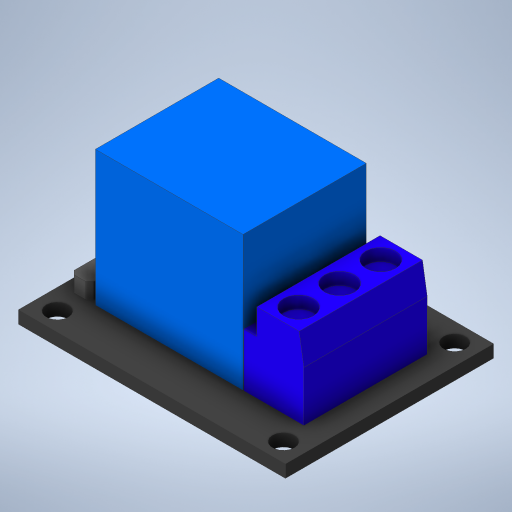
# Autodesk Inventor part: 릴레이모듈
Saved by Autodesk Inventor 2023 (Build 270158000, 158)
## iProperties
Created: 2022-06-23
Part Number: 릴레이모듈
Material: 일반
Document SubType Name: Modeling
Designer: user
Density: 1 g/cm^3
Appearance: 기본값
Author: user
Autodesk Inventor part; units mm, degrees
ref_plane "YZ Plane" through (0, 0, 0) normal (1, 0, 0) x (0, 1, 0)
ref_plane "XZ Plane" through (0, 0, 0) normal (0, 1, 0) x (-1, 0, 0)
ref_plane "XY Plane" through (0, 0, 0) normal (0, 0, 1) x (1, 0, 0)
sketch "스케치1" plane through (0, 0, 0) normal (0, 0, 1) x (1, 0, 0)
  line L0 (-17, 13.25) -> (17, 13.25)
  line L1 (17, 13.25) -> (17, -13.25)
  line L2 (17, -13.25) -> (-17, -13.25)
  line L3 (-17, -13.25) -> (-17, 13.25)
  line L4 (-17, 13.25) -> (17, -13.25) construction
  line L5 (17, 13.25) -> (-17, -13.25) construction
  circle A0 centre (14.4, 10.9) radius 1.4
  line L6 (0, 0) -> (4.1971, 0)
  line L7 (0, 0) -> (0, 5.4603)
  circle A1 centre (-14.4, 10.9) radius 1.4
  circle A2 centre (14.4, -10.9) radius 1.4
  circle A3 centre (-14.4, -10.9) radius 1.4
  dimension "d0" = 34
  dimension "d1" = 26.5
  dimension "d2" = 28.8
  dimension "d3" = 2.8
  dimension "d4" = 21.8
  constraints: 16 end point, 4 centre point, 3 symmetric about line, 2 horizontal, 2 midpoint, 2 parallel, 1 perpendicular, 1 vertical, 3 other
  measures "d0" distance of L1.end L2.end
  measures "d1" distance of L0.end L1.end
  measures "d2" distance of A0.centre A1.centre
  measures "d3" diameter of A0
  measures "d4" distance of A2.centre A0.centre
extrude "돌출1" add sketch "스케치1" along normal blind 1.6
sketch "스케치2" plane through (0, 0, 1.6) normal (0, 0, 1) x (1, 0, 0)
  line L0 (12.6, -7.85) -> (-6.2, -7.85)
  line L1 (-6.2, -7.85) -> (-6.2, 7.85)
  line L2 (-6.2, 7.85) -> (12.6, 7.85)
  line L3 (12.6, 7.85) -> (12.6, -7.85)
  line L4 (12.6, -7.85) -> (-6.2, 7.85) construction
  line L5 (-6.2, -7.85) -> (12.6, 7.85) construction
  line L6 (17, -13.25) -> (17, 13.25) projected
  point P0 (0, 0)
  point P1 (3.2, 0)
  dimension "d7" = 15.7
  dimension "d8" = 18.8
  dimension "d9" = 4.4
  constraints: 12 end point, 2 midpoint, 2 parallel, 1 horizontal, 1 perpendicular
  measures "d7" distance of L2.end L0.start
  measures "d8" distance of L0.start L0.end
  measures "d9" distance between parallel lines of L6 L3
extrude "돌출2" add sketch "스케치2" along normal blind 17.2
sketch "스케치3" plane through (-6.2, 7.85, 1.6) normal (0, 1, 0) x (1, 0, 0)
  line L0 (0, 0) -> (18.8, 0) projected
  line L1 (0, 0) -> (-1.75, 0)
  line L2 (-1.75, 0) -> (-1.75, -6.84)
  line L3 (-1.75, -6.84) -> (0, -6.84)
  line L4 (0, -6.84) -> (0, 0)
  line L5 (-1.75, 0) -> (-7.75, 0)
  line L6 (-7.75, 0) -> (-7.75, -10.1)
  line L7 (-7.75, -10.1) -> (-1.75, -10.1)
  line L8 (-1.75, -10.1) -> (-1.75, 0)
  line L9 (-7.15, -10.1) -> (-7.75, -6.4)
  line L10 (-0.1, -6.84) -> (-0.1, 0)
  line L11 (23.2, 0) -> (-10.8, 0) projected
  point P0 (6.2, 1.6)
  point P1 (-1.75, -6.84)
  dimension "d12" = 1.75
  dimension "d13" = 6.84
  dimension "d14" = 6
  dimension "d15" = 10.1
  dimension "d16" = 0.6
  dimension "d17" = 3.7
  dimension "d20" = 0.1
  constraints: 20 end point, 4 parallel, 4 point on line, 3 perpendicular, 2 horizontal
  measures "d12" distance of L3.end L2.end
  measures "d13" distance of L2.end L1.end
  measures "d14" distance of L6.end L7.end
  measures "d15" distance of L5.end L6.end
  measures "d16" distance of L6.end L9.start
  measures "d17" distance of L6.end L9.end
  measures "d20" distance between parallel lines of L4 L10
extrude "돌출3" add sketch "스케치3" against normal blind 15.7 contours L10 L3 L2 L1 | L2 L8 L7 L9 L6 L5
sketch "스케치4" plane through (-13.35, 7.85, 11.7) normal (0, 0, 1) x (1, 0, 0)
  line L0 (0, 0) -> (5.4, 0) projected
  line L1 (0, 0) -> (0, -15.7) projected
  line L2 (5.4, -15.7) -> (0, -15.7) projected
  line L3 (5.4, 0) -> (5.4, -15.7) projected
  line L4 (5.4, 0) -> (5.4, -15.7) projected
  line L5 (5.4, -7.85) -> (0, -7.85)
  circle A0 centre (2.7, -7.85) radius 1.9
  circle A1 centre (2.7, -13.0833) radius 1.9
  circle A2 centre (2.7, -2.6167) radius 1.9
  circle A3 centre (2.7, -7.85) radius 1.9
  point P0 (13.35, -7.85)
  dimension "d21" = 3.8
  dimension "d24" = 5.2333
  dimension "d27" = 5.2333
  constraints: 4 centre point, 3 midpoint, 2 end point, 2 vertical, 6 other
  measures "d21" diameter of A0
  measures "d24" distance of A0.centre A1.centre
  measures "d27" distance of A0.centre A2.centre
extrude "돌출4" cut sketch "스케치4" against normal blind 1.54 contours A0 L5 | L5 A0 | A1 | A2
sketch "스케치5" plane through (0, 0, 1.6) normal (0, 0, 1) x (1, 0, 0)
  line L0 (15.8, 7.85) -> (13.3, 7.85)
  line L1 (13.3, 7.85) -> (13.3, 0.4)
  line L2 (13.3, 0.4) -> (15.8, 0.4)
  line L3 (15.8, 0.4) -> (15.8, 7.85)
  line L4 (17, -13.25) -> (17, 13.25) projected
  point P0 (0, 0)
  dimension "d32" = 2.5
  dimension "d33" = 7.45
  dimension "d34" = 1.2
  constraints: 8 end point, 2 parallel, 1 horizontal, 1 perpendicular
  measures "d32" distance of L2.end L1.end
  measures "d33" distance of L1.end L0.end
  measures "d34" distance between parallel lines of L4 L3
extrude "돌출5" add sketch "스케치5" along normal blind 2
chamfer "모따기1" distance 0.5 angle 45 4 edges at (15.8, 7.85, 2.6) (15.8, 0.4, 2.6) (13.3, 7.85, 2.6) (13.3, 0.4, 2.6)
